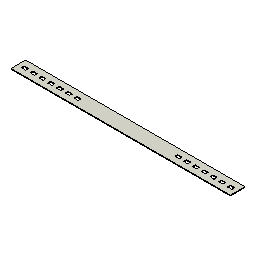
rubber_band (Autodesk Fusion 360 design; units mm, degrees)
Autodesk Fusion 360 part; units mm, degrees
sketch "Sketch2" plane through (0, 0, 0) normal (0, 0, 1) x (1, 0, 0)
  line L0 (-150, 10) -> (150, 10)
  line L1 (150, 10) -> (150, -10)
  line L2 (150, -10) -> (-150, -10)
  line L3 (-150, -10) -> (-150, 10)
  line L4 (0, 10) -> (0, -10) construction
  line L5 (-150, 2) -> (150, 2) construction
  line L6 (150, -2) -> (-150, -2) construction
  line L7 (-143.5, 2) -> (-138.5, 2)
  line L8 (-138, 1.5) -> (-138, -1.5)
  line L9 (-138.5, -2) -> (-143.5, -2)
  line L10 (-144, -1.5) -> (-144, 1.5)
  arc A0 (-143.5, 2) -> (-144, 1.5) centre (-143.5, 1.5) ccw
  arc A1 (-138, 1.5) -> (-138.5, 2) centre (-138.5, 1.5) ccw
  arc A2 (-138.5, -2) -> (-138, -1.5) centre (-138.5, -1.5) ccw
  arc A3 (-144, -1.5) -> (-143.5, -2) centre (-143.5, -1.5) ccw
  arc A4 (-132, -1.5) -> (-131.5, -2) centre (-131.5, -1.5) ccw
  line L11 (-132, -1.5) -> (-132, 1.5)
  arc A5 (-131.5, 2) -> (-132, 1.5) centre (-131.5, 1.5) ccw
  line L12 (-131.5, 2) -> (-126.5, 2)
  arc A6 (-126, 1.5) -> (-126.5, 2) centre (-126.5, 1.5) ccw
  line L13 (-126, 1.5) -> (-126, -1.5)
  arc A7 (-126.5, -2) -> (-126, -1.5) centre (-126.5, -1.5) ccw
  line L14 (-126.5, -2) -> (-131.5, -2)
  arc A8 (-120, -1.5) -> (-119.5, -2) centre (-119.5, -1.5) ccw
  line L15 (-120, -1.5) -> (-120, 1.5)
  arc A9 (-119.5, 2) -> (-120, 1.5) centre (-119.5, 1.5) ccw
  line L16 (-119.5, 2) -> (-114.5, 2)
  arc A10 (-114, 1.5) -> (-114.5, 2) centre (-114.5, 1.5) ccw
  line L17 (-114, 1.5) -> (-114, -1.5)
  arc A11 (-114.5, -2) -> (-114, -1.5) centre (-114.5, -1.5) ccw
  line L18 (-114.5, -2) -> (-119.5, -2)
  arc A12 (-108, -1.5) -> (-107.5, -2) centre (-107.5, -1.5) ccw
  line L19 (-108, -1.5) -> (-108, 1.5)
  arc A13 (-107.5, 2) -> (-108, 1.5) centre (-107.5, 1.5) ccw
  line L20 (-107.5, 2) -> (-102.5, 2)
  arc A14 (-102, 1.5) -> (-102.5, 2) centre (-102.5, 1.5) ccw
  line L21 (-102, 1.5) -> (-102, -1.5)
  arc A15 (-102.5, -2) -> (-102, -1.5) centre (-102.5, -1.5) ccw
  line L22 (-102.5, -2) -> (-107.5, -2)
  arc A16 (-96, -1.5) -> (-95.5, -2) centre (-95.5, -1.5) ccw
  line L23 (-96, -1.5) -> (-96, 1.5)
  arc A17 (-95.5, 2) -> (-96, 1.5) centre (-95.5, 1.5) ccw
  line L24 (-95.5, 2) -> (-90.5, 2)
  arc A18 (-90, 1.5) -> (-90.5, 2) centre (-90.5, 1.5) ccw
  line L25 (-90, 1.5) -> (-90, -1.5)
  arc A19 (-90.5, -2) -> (-90, -1.5) centre (-90.5, -1.5) ccw
  line L26 (-90.5, -2) -> (-95.5, -2)
  arc A20 (-84, -1.5) -> (-83.5, -2) centre (-83.5, -1.5) ccw
  line L27 (-84, -1.5) -> (-84, 1.5)
  arc A21 (-83.5, 2) -> (-84, 1.5) centre (-83.5, 1.5) ccw
  line L28 (-83.5, 2) -> (-78.5, 2)
  arc A22 (-78, 1.5) -> (-78.5, 2) centre (-78.5, 1.5) ccw
  line L29 (-78, 1.5) -> (-78, -1.5)
  arc A23 (-78.5, -2) -> (-78, -1.5) centre (-78.5, -1.5) ccw
  line L30 (-78.5, -2) -> (-83.5, -2)
  arc A24 (-72, -1.5) -> (-71.5, -2) centre (-71.5, -1.5) ccw
  line L31 (-72, -1.5) -> (-72, 1.5)
  arc A25 (-71.5, 2) -> (-72, 1.5) centre (-71.5, 1.5) ccw
  line L32 (-71.5, 2) -> (-66.5, 2)
  arc A26 (-66, 1.5) -> (-66.5, 2) centre (-66.5, 1.5) ccw
  line L33 (-66, 1.5) -> (-66, -1.5)
  arc A27 (-66.5, -2) -> (-66, -1.5) centre (-66.5, -1.5) ccw
  line L34 (-66.5, -2) -> (-71.5, -2)
  arc A28 (84, 1.5) -> (83.5, 2) centre (83.5, 1.5) ccw
  line L35 (90, 1.5) -> (90, -1.5)
  line L36 (78, 1.5) -> (78, -1.5)
  arc A29 (78, -1.5) -> (78.5, -2) centre (78.5, -1.5) ccw
  arc A30 (90, -1.5) -> (90.5, -2) centre (90.5, -1.5) ccw
  line L37 (83.5, 2) -> (78.5, 2)
  line L38 (84, -1.5) -> (84, 1.5)
  arc A31 (90.5, 2) -> (90, 1.5) centre (90.5, 1.5) ccw
  arc A32 (83.5, -2) -> (84, -1.5) centre (83.5, -1.5) ccw
  arc A33 (78.5, 2) -> (78, 1.5) centre (78.5, 1.5) ccw
  line L39 (78.5, -2) -> (83.5, -2)
  line L40 (138.5, -2) -> (143.5, -2)
  line L41 (144, -1.5) -> (144, 1.5)
  arc A34 (66.5, 2) -> (66, 1.5) centre (66.5, 1.5) ccw
  line L42 (71.5, 2) -> (66.5, 2)
  arc A35 (71.5, -2) -> (72, -1.5) centre (71.5, -1.5) ccw
  line L43 (72, -1.5) -> (72, 1.5)
  arc A36 (138.5, 2) -> (138, 1.5) centre (138.5, 1.5) ccw
  line L44 (66, 1.5) -> (66, -1.5)
  arc A37 (72, 1.5) -> (71.5, 2) centre (71.5, 1.5) ccw
  arc A38 (144, 1.5) -> (143.5, 2) centre (143.5, 1.5) ccw
  arc A39 (143.5, -2) -> (144, -1.5) centre (143.5, -1.5) ccw
  arc A40 (138, -1.5) -> (138.5, -2) centre (138.5, -1.5) ccw
  line L45 (138, 1.5) -> (138, -1.5)
  line L46 (143.5, 2) -> (138.5, 2)
  arc A41 (66, -1.5) -> (66.5, -2) centre (66.5, -1.5) ccw
  line L47 (66.5, -2) -> (71.5, -2)
  line L48 (90.5, -2) -> (95.5, -2)
  arc A42 (96, 1.5) -> (95.5, 2) centre (95.5, 1.5) ccw
  line L49 (102.5, -2) -> (107.5, -2)
  line L50 (102, 1.5) -> (102, -1.5)
  arc A43 (102.5, 2) -> (102, 1.5) centre (102.5, 1.5) ccw
  arc A44 (107.5, -2) -> (108, -1.5) centre (107.5, -1.5) ccw
  line L51 (96, -1.5) -> (96, 1.5)
  line L52 (95.5, 2) -> (90.5, 2)
  arc A45 (102, -1.5) -> (102.5, -2) centre (102.5, -1.5) ccw
  line L53 (108, -1.5) -> (108, 1.5)
  arc A46 (108, 1.5) -> (107.5, 2) centre (107.5, 1.5) ccw
  arc A47 (95.5, -2) -> (96, -1.5) centre (95.5, -1.5) ccw
  line L54 (107.5, 2) -> (102.5, 2)
  line L55 (114, 1.5) -> (114, -1.5)
  line L56 (119.5, 2) -> (114.5, 2)
  arc A48 (120, 1.5) -> (119.5, 2) centre (119.5, 1.5) ccw
  arc A49 (119.5, -2) -> (120, -1.5) centre (119.5, -1.5) ccw
  arc A50 (114.5, 2) -> (114, 1.5) centre (114.5, 1.5) ccw
  arc A51 (114, -1.5) -> (114.5, -2) centre (114.5, -1.5) ccw
  arc A52 (132, 1.5) -> (131.5, 2) centre (131.5, 1.5) ccw
  line L57 (131.5, 2) -> (126.5, 2)
  arc A53 (126.5, 2) -> (126, 1.5) centre (126.5, 1.5) ccw
  line L58 (126, 1.5) -> (126, -1.5)
  line L59 (120, -1.5) -> (120, 1.5)
  arc A54 (131.5, -2) -> (132, -1.5) centre (131.5, -1.5) ccw
  arc A55 (126, -1.5) -> (126.5, -2) centre (126.5, -1.5) ccw
  line L60 (126.5, -2) -> (131.5, -2)
  line L61 (114.5, -2) -> (119.5, -2)
  line L62 (132, -1.5) -> (132, 1.5)
  point P0 (-150, 0)
  point P1 (-144, 2)
  point P2 (-138, 2)
  point P3 (144, 2)
  point P4 (138, 2)
  dimension "d32" = 300
  dimension "d33" = 20
  dimension "d34" = 2
  dimension "d35" = 2
  dimension "d36" = 6
  dimension "d37" = 6
  dimension "d39" = 0.5
  dimension "d42" = 12
  dimension "d43" = 0
  constraint horizontal L0
  constraint vertical L1
  constraint horizontal L2
  constraint vertical L3
  constraint midpoint L0 L4.start
  constraint midpoint L2 L4.end
  constraint midpoint origin L4
  constraint coincident L3 L5.start
  constraint coincident L1 L5.end
  constraint perpendicular L1 L5
  constraint coincident L1 L6.start
  constraint coincident L3 L6.end
  constraint perpendicular L3 L6
  constraint midpoint L3 P0
  constraint horizontal L7
  constraint vertical L8
  constraint horizontal L9
  constraint vertical L10
  constraint coincident L5 P1
  constraint coincident P1 L7
  constraint coincident P1 L10
  constraint tangent L7 A0
  constraint tangent L10 A0
  constraint coincident P2 L7
  constraint coincident P2 L8
  constraint tangent L7 A1
  constraint tangent L8 A1
  constraint equal A0 A1
  constraint tangent L8 A2
  constraint tangent L9 A2
  constraint equal A0 A2
  constraint tangent L9 A3
  constraint tangent L10 A3
  constraint equal A0 A3
  constraint coincident L6 L9.start
  constraint symmetric L4 P1 P3
  constraint symmetric L4 P2 P4
  constraint symmetric L4 L7.start A38.end
  constraint symmetric L4 L10.end L41.end
  constraint symmetric L4 A0 A38
  constraint symmetric L4 L7.end A36.start
  constraint symmetric L4 L8.start A36.end
  constraint symmetric L4 A1 A36
  constraint symmetric L4 L8.end A40.start
  constraint symmetric L4 L9.start L40.start
  constraint symmetric L4 A2 A40
  constraint symmetric L4 L9.end L40.end
  constraint symmetric L4 L10.start L41.start
  constraint symmetric L4 A3 A39
  constraint symmetric L4 A4.start A54.end
  constraint symmetric L4 A4.end A54.start
  constraint symmetric L4 A4 A54
  constraint symmetric L4 L11.end A52.start
  constraint symmetric L4 A5.start A52.end
  constraint symmetric L4 A5 A52
  constraint symmetric L4 L12.end L57.end
  constraint symmetric L4 A6.start A53.end
  constraint symmetric L4 A6 A53
  constraint symmetric L4 L13.end L58.end
  constraint symmetric L4 A7.start A55.end
  constraint symmetric L4 A7 A55
  constraint symmetric L4 A8.start A49.end
  constraint symmetric L4 A8.end A49.start
  constraint symmetric L4 A8 A49
  constraint symmetric L4 L15.end A48.start
  constraint symmetric L4 A9.start L56.start
  constraint symmetric L4 A9 A48
  constraint symmetric L4 L16.end L56.end
  constraint symmetric L4 A10.start L55.start
  constraint symmetric L4 A10 A50
  constraint symmetric L4 L17.end L55.end
  constraint symmetric L4 A11.start A51.end
  constraint symmetric L4 A11 A51
  constraint symmetric L4 A12.start A44.end
  constraint symmetric L4 A12.end L49.end
  constraint symmetric L4 A12 A44
  constraint symmetric L4 L19.end L53.end
  constraint symmetric L4 A13.start A46.end
  constraint symmetric L4 A13 A46
  constraint symmetric L4 L20.end A43.start
  constraint symmetric L4 A14.start L50.start
  constraint symmetric L4 A14 A43
  constraint symmetric L4 L21.end L50.end
  constraint symmetric L4 A15.start L49.start
  constraint symmetric L4 A15 A45
  constraint symmetric L4 A16.start L51.start
  constraint symmetric L4 A16.end L48.end
  constraint symmetric L4 A16 A47
  constraint symmetric L4 L23.end A42.start
  constraint symmetric L4 A17.start A42.end
  constraint symmetric L4 A17 A42
  constraint symmetric L4 L24.end A31.start
  constraint symmetric L4 A18.start L35.start
  constraint symmetric L4 A18 A31
  constraint symmetric L4 L25.end L35.end
  constraint symmetric L4 A19.start A30.end
  constraint symmetric L4 A19 A30
  constraint symmetric L4 A20.start L38.start
  constraint symmetric L4 A20.end A32.start
  constraint symmetric L4 A20 A32
  constraint symmetric L4 L27.end A28.start
  constraint symmetric L4 A21.start A28.end
  constraint symmetric L4 A21 A28
  constraint symmetric L4 L28.end L37.end
  constraint symmetric L4 A22.start L36.start
  constraint symmetric L4 A22 A33
  constraint symmetric L4 L29.end L36.end
  constraint symmetric L4 A23.start A29.end
  constraint symmetric L4 A23 A29
  constraint symmetric L4 A24.start A35.end
  constraint symmetric L4 A24.end A35.start
  constraint symmetric L4 A24 A35
  constraint symmetric L4 L31.end L43.end
  constraint symmetric L4 A25.start L42.start
  constraint symmetric L4 A25 A37
  constraint symmetric L4 L32.end A34.start
  constraint symmetric L4 A26.start A34.end
  constraint symmetric L4 A26 A34
  constraint symmetric L4 L33.end L44.end
  constraint symmetric L4 A27.start A41.end
  constraint symmetric L4 A27 A41
  measures "d32" distance of L0.start L0.end
  measures "d33" distance of L0.start L2.end
  measures "d34" distance of L6 P0
  measures "d35" distance of L5.start P0
  measures "d36" distance of L3 L10
  measures "d37" distance of P1 P2
  measures "d39" radius of A0
extrude "Extrude1" add sketch "Sketch2" along normal blind 1
